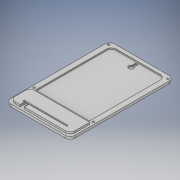
# Autodesk Inventor part: Top
Saved by Autodesk Inventor 2019 (Build 230136000, 136)
## iProperties
Created: 2020-07-22
Part Number: Top
Material: Generic
Document SubType Name: Modeling
Designer: Erle
Density: 1 g/cm^3
Appearance: Default
Author: Erle
Autodesk Inventor part; units mm, degrees
ref_plane "YZ Plane" through (0, 0, 0) normal (1, 0, 0) x (0, 1, 0)
ref_plane "XZ Plane" through (0, 0, 0) normal (0, 1, 0) x (-1, 0, 0)
ref_plane "XY Plane" through (0, 0, 0) normal (0, 0, 1) x (1, 0, 0)
sketch "Sketch1" plane through (0, 0, 0) normal (0, 1, 0) x (-1, 0, 0)
  line L0 (52.5, 85) -> (-52.5, 85)
  line L1 (-52.5, 85) -> (-52.5, -85)
  line L2 (-52.5, -85) -> (52.5, -85)
  line L3 (52.5, -85) -> (52.5, 85)
  line L4 (52.5, 85) -> (-52.5, -85) construction
  line L5 (-52.5, 85) -> (52.5, -85) construction
  point P0 (0, 0)
  dimension "d0" = 170
  dimension "d1" = 105
  constraints: 12 end point, 2 midpoint, 2 parallel, 1 horizontal, 1 perpendicular
  measures "d0" distance of L2.end L0.start
  measures "d1" distance of L1.end L2.end
extrude "Extrusion1" add sketch "Sketch1" along normal blind 4
sketch "Sketch2" plane through (0, 4, 0) normal (0, 1, 0) x (1, 0, 0)
  line L0 (-44, 79) -> (44, 79)
  line L1 (44, 79) -> (44, -45)
  line L2 (44, -45) -> (-44, -45)
  line L3 (-44, -45) -> (-44, 79)
  line L4 (52.5, 85) -> (-52.5, 85) projected
  point P0 (0, 0)
  point P1 (0, 79)
  dimension "d4" = 124
  dimension "d5" = 88
  dimension "d6" = 6
  constraints: 8 end point, 2 parallel, 1 horizontal, 1 midpoint, 1 perpendicular, 1 vertical alignment
  measures "d4" distance of L2.end L0.start
  measures "d5" distance of L0.start L0.end
  measures "d6" distance between parallel lines of L4 L0
extrude "Extrusion2" cut sketch "Sketch2" against normal blind 2
sketch "Sketch3" plane through (0, 4, 0) normal (0, 1, 0) x (1, 0, 0)
  line L0 (-49, -49.5) -> (49, -49.5)
  line L1 (49, -49.5) -> (49, -81.5)
  line L2 (49, -81.5) -> (-49, -81.5)
  line L3 (-49, -81.5) -> (-49, -49.5)
  line L4 (-52.5, 85) -> (-52.5, -85) projected
  line L5 (-52.5, -85) -> (52.5, -85) projected
  point P0 (0, 0)
  point P1 (0, -49.5)
  dimension "d9" = 3.5
  dimension "d10" = 3.5
  dimension "d11" = 32
  constraints: 8 end point, 2 parallel, 1 horizontal, 1 midpoint, 1 perpendicular, 1 vertical alignment
  measures "d9" distance between parallel lines of L4 L3
  measures "d10" distance between parallel lines of L5 L2
  measures "d11" distance of L2.end L0.start
extrude "Extrusion3" add sketch "Sketch3" along normal blind 3
fillet "Fillet1" radius 8 9 edges at (52.5, 2, 85) (-52.5, 2, 85) (52.5, 2, -85) (-52.5, 2, -85) (-44, 3, -79) (44, 3, -79) (-49, 5.5, 49.5) (-49, 5.5, 81.5) (49, 5.5, 81.5)
sketch "Sketch4" plane through (0, 0, 0) normal (0, -1, 0) x (1, 0, 0)
  line L0 (48.5, -79) -> (-48.5, -79) construction
  line L1 (-48.5, -79) -> (-48.5, 43) construction
  line L2 (-48.5, 43) -> (48.5, 43) construction
  line L3 (48.5, 43) -> (48.5, -79) construction
  line L4 (52.5, 77) -> (52.5, -77) projected
  line L5 (44.5, -85) -> (-44.5, -85) construction
  point P0 (0, 0)
  point P1 (0, -79)
  dimension "d15" = 4
  dimension "d16" = 122
  dimension "d17" = 6
  constraints: 8 end point, 4 coincident, 2 parallel, 1 horizontal, 1 midpoint, 1 perpendicular, 1 vertical alignment
  measures "d15" distance between parallel lines of L4 L3
  measures "d16" distance of L2.end L0.start
  measures "d17" distance between parallel lines of L5 L0
hole "Hole1" at (48.5, 0, -79) at (-48.5, 0, -79) at (-48.5, 0, 43) at (48.5, 0, 43) direction (0, 1, 0) diameter 3.4 depth 8 tip angle 118 countersink diameter 6.3 countersink angle 90 clearance for "Countersunk Flat Head Screw DIN EN ISO 2009" size "M3" standard "DIN"
sketch "Sketch5" plane through (0, 2, 0) normal (0, 1, 0) x (1, 0, 0)
  arc A0 (-2, 71) -> (2, 71) centre (0, 67.5359) ccw
  line L0 (-2, 71) -> (-2, 77)
  line L1 (-2, 77) -> (2, 77)
  line L2 (2, 77) -> (2, 71)
  line L3 (-36, 79) -> (36, 79) projected
  point P0 (0, 0)
  point P1 (0, 77)
  dimension "d25" = 4
  dimension "d26" = 4
  dimension "d27" = 6
  dimension "d28" = 2
  constraints: 6 end point, 2 perpendicular, 2 point on circle, 2 vertical alignment, 1 centre point, 1 midpoint, 1 vertical
  measures "d25" radius of A0
  measures "d26" distance of L0.end L1.end
  measures "d27" distance of L1.end L2.end
  measures "d28" distance from line of L3 point (0, 77)
extrude "Extrusion4" cut sketch "Sketch5" against normal blind 10
sketch "Sketch6" plane through (0, 7, 0) normal (0, 1, 0) x (1, 0, 0)
  line L0 (-41, -81.5) -> (41, -81.5) projected
  line L1 (-33.15, -81.5) -> (-26.15, -81.5)
  line L2 (-26.15, -81.5) -> (-26.15, -75)
  line L3 (-26.15, -75) -> (-33.15, -75)
  line L4 (-33.15, -75) -> (-33.15, -81.5)
  line L5 (-49, -57.5) -> (-49, -73.5) projected
  point P0 (0, 0)
  dimension "d31" = 15.85
  dimension "d32" = 7
  dimension "d33" = 6.5
  constraints: 8 end point, 2 parallel, 1 horizontal, 1 perpendicular, 1 point on line
  measures "d31" distance between parallel lines of L4 L5
  measures "d32" distance of L2.end L3.end
  measures "d33" distance of L1.end L2.end
extrude "Extrusion5" cut sketch "Sketch6" against normal up to surface (3 mm away)
sketch "Sketch7" plane through (0, 7, 0) normal (0, 1, 0) x (1, 0, 0)
  line L0 (-36, -74) -> (36, -74)
  line L1 (36, -74) -> (36, -72)
  line L2 (36, -72) -> (-36, -72)
  line L3 (-36, -72) -> (-36, -74)
  line L4 (-26.15, -81.5) -> (41, -81.5) projected
  point P0 (0, 0)
  point P1 (0, -72)
  dimension "d36" = 72
  dimension "d37" = 2
  dimension "d38" = 7.5
  constraints: 8 end point, 2 parallel, 1 horizontal, 1 midpoint, 1 perpendicular, 1 vertical alignment
  measures "d36" distance of L1.end L2.end
  measures "d37" distance of L0.end L1.end
  measures "d38" distance between parallel lines of L4 L0
extrude "Extrusion6" cut sketch "Sketch7" against normal blind 2
body "Solid1"
